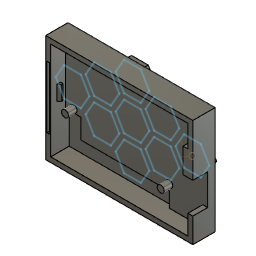
Arduino Pro Holder v8 (Autodesk Fusion 360 design; units mm, degrees)
Autodesk Fusion 360 part; units mm, degrees
sketch "Arduino" plane through (0, 0, 0) normal (0, 0, 1) x (1, 0, 0)
  line L0 (0, 0) -> (54.5, 0)
  line L1 (54.5, 0) -> (54.5, 38.5)
  line L2 (54.5, 38.5) -> (0, 38.5)
  line L3 (0, 38.5) -> (0, 0)
  circle A0 centre (41.5, 8) radius 1.75
  circle A1 centre (2.8, 15) radius 1.75
  line L4 (54.5, 19) -> (48.5, 19)
  line L5 (48.5, 19) -> (48.5, 9)
  line L6 (48.5, 9) -> (54.5, 9)
  line L7 (54.5, 9) -> (54.5, 19)
  dimension "d1" = 54.5
  dimension "d2" = 38.5
  dimension "d3" = 3.5
  dimension "d4" = 3.5
  dimension "d5" = 13
  dimension "d6" = 8
  dimension "d7" = 15
  dimension "d8" = 2.8
  dimension "d9" = 6
  dimension "d10" = 10
  dimension "d11" = 9
  constraint horizontal L0
  constraint vertical L1
  constraint horizontal L2
  constraint vertical L3
  constraint coincident L0.start L3.end
  constraint horizontal L4
  constraint vertical L5
  constraint horizontal L6
  constraint vertical L7
  constraint coincident L1 L4.start
  measures "d1" distance of L0.start L0.end
  measures "d2" distance of L0.start L2.end
  measures "d3" diameter of A0
  measures "d4" diameter of A1
  measures "d5" distance of L1 A0.centre
  measures "d6" distance of L0 A0.centre
  measures "d7" distance of L0 A1.centre
  measures "d8" distance of L3 A1.centre
  measures "d9" distance of L4.start L4.end
  measures "d10" distance of L4.start L6.end
  measures "d11" distance of L0 L6
sketch "Shell Outline" plane through (0, 0, 0) normal (0, 0, 1) x (1, 0, 0)
  circle A0 centre (-0.6853, 15.304) radius 1.4
  circle A1 centre (38.0147, 8.304) radius 1.4
  line L0 (51.5147, 39.304) -> (-3.9853, 39.304)
  line L1 (-3.9853, 39.304) -> (-3.9853, -0.196)
  line L2 (-3.9853, -0.196) -> (51.5147, -0.196)
  line L3 (51.5147, -0.196) -> (51.5147, 39.304)
  line L4 (-5.9853, -2.196) -> (53.5147, -2.196)
  line L5 (53.5147, -2.196) -> (53.5147, 41.304)
  line L6 (53.5147, 41.304) -> (-5.9853, 41.304)
  line L7 (-5.9853, 41.304) -> (-5.9853, -2.196)
  line L8 (51.0147, 20.304) -> (53.5147, 20.304)
  line L9 (53.5147, 20.304) -> (53.5147, 7.804)
  line L10 (53.5147, 7.804) -> (51.0147, 7.804)
  line L11 (51.5147, 39.304) -> (-3.9853, 39.304)
  line L12 (-3.9853, 39.304) -> (-3.9853, 33.304)
  line L13 (-3.9853, 33.304) -> (51.5147, 33.304)
  line L14 (51.5147, 33.304) -> (51.5147, 39.304)
  line L15 (-3.9853, -0.196) -> (38.0147, -0.196)
  line L16 (38.0147, -0.196) -> (38.0147, 5.804)
  line L17 (38.0147, 5.804) -> (-3.9853, 5.804)
  line L18 (-3.9853, 5.804) -> (-3.9853, -0.196)
  line L19 (-3.9853, 5.804) -> (2.259, 5.804)
  line L20 (2.259, 5.804) -> (2.259, 13.804)
  line L21 (2.259, 13.804) -> (-3.9853, 13.804)
  line L22 (-3.9853, 13.804) -> (-3.9853, 5.804)
  point P0 (-3.4853, 0.304)
  dimension "d16" = 2.8
  dimension "d17" = 2.8
  dimension "d33" = 12.5
  dimension "d34" = 8
  dimension "d36" = 2
  dimension "d37" = 6
  dimension "d38" = 42
  dimension "d39" = 6
  dimension "d40" = 8
  constraint horizontal L8
  constraint vertical L9
  constraint coincident L5 L9.end
  constraint horizontal L11
  constraint vertical L12
  constraint horizontal L13
  constraint vertical L14
  constraint horizontal L15
  constraint vertical L16
  constraint horizontal L17
  constraint vertical L18
  constraint horizontal L19
  constraint vertical L20
  constraint horizontal L21
  constraint vertical L22
  measures "d16" diameter of A1
  measures "d17" diameter of A0
  measures "d33" distance of L8 L10
  measures "d34" distance of L2 L10
  measures "d36" distance of L2 L4
  measures "d37" distance of L0.start L13.end
  measures "d38" distance of L1.end L15.end
  measures "d39" distance of L1.end L17.end
  measures "d40" distance of L17.end L21.end
extrude "Extrude1" add sketch "Arduino" along normal blind 6 contours L0 L1 L2 L3 L4 L5 L6 makes body 1
move_body "Move1" bodies 1 to x (1, 0, 0) y (0, 1, 0) z (0, 0, 1) at (-3, 0, 0)
move_body "Move2" bodies 1 to x (1, 0, 0) y (0, 1, 0) z (0, 0, 1) at (-0.4853, 0.304, 0)
extrude "Extrude2" add sketch "Shell Outline" against normal blind 2 separate body contours A0 | A1 | L0 L1 L3 L11 L12 L13 L14 | L0 L1 L2 L3 L4 L5 L6 L7 L8 L10 L11 L12 L14 L15 L18 L22 | L1 L2 L3 L13 L16 L17 L20 L21 | L3 L5 L8 L9 L10 | L1 L17 L19 L20 L21 L22 | L1 L2 L15 L16 L17 L18 L19 makes body 2
extrude "Extrude3" add sketch "Shell Outline" along normal blind 3.5 separate body contours A0 | A1 makes body 3 at (37.9798, 9.7036, 2.3333) makes body 4 at (0.7077, 15.1646, 2.3333)
extrude "Extrude4" add sketch "Shell Outline" along normal blind 6 separate body contours L0 L1 L2 L3 L4 L5 L6 L7 L8 L10 L11 L12 L14 L15 L18 L22 makes body 5
combine "Combine1" operation add target body 2 tool bodies 3 4 5
extrude "Extrude5" cut sketch "Shell Outline" against normal blind 1.5 contours L0 L1 L3 L11 L12 L13 L14 | L1 L17 L19 L20 L21 L22 | L1 L2 L15 L16 L17 L18 L19 bodies 2
extrude "Extrude6" add 1 faces at (33.6814, 26.804, -2) along direction (0, 0, -1) blind 1 on bodies 2 bodies 2
sketch "Sketch3" plane through (51.5147, 0, 0) normal (-1, 0, 0) x (0, 0, 1)
  line L0 (0, 33.304) -> (0, 20.304)
  line L1 (0, 20.304) -> (6, 20.304)
  line L2 (6, 20.304) -> (6, 39.304)
  line L3 (6, 39.304) -> (-1.5, 39.304)
  line L4 (-1.5, 39.304) -> (-1.5, 33.304)
  line L5 (-1.5, 33.304) -> (0, 33.304)
  line L6 (6, 20.304) -> (3, 20.304)
  line L7 (3, 20.304) -> (3, 30.304)
  line L8 (3, 30.304) -> (6, 30.304)
  line L9 (6, 30.304) -> (6, 20.304)
  dimension "d45" = 10
  constraint horizontal L6
  constraint vertical L7
  constraint horizontal L8
  constraint vertical L9
  constraint coincident L1.end L2.start
  measures "d45" distance of L1.end L8.end
extrude "Extrude7" add sketch "Sketch3" along normal blind 2 contours L1 L2 L6 L7 L8 L9 bodies 2
sketch "Sketch4" plane through (-3.9853, 0, 0) normal (1, 0, 0) x (0, 0, -1)
  line L0 (1.5, 39.304) -> (-6, 39.304)
  line L1 (-6, 39.304) -> (-6, -0.196)
  line L2 (-6, -0.196) -> (1.5, -0.196)
  line L3 (1.5, -0.196) -> (1.5, 13.804)
  line L4 (1.5, 13.804) -> (0, 13.804)
  line L5 (0, 13.804) -> (0, 33.304)
  line L6 (0, 33.304) -> (1.5, 33.304)
  line L7 (1.5, 33.304) -> (1.5, 39.304)
  line L8 (-2, 36) -> (-2, 7) construction
  line L9 (-2, 18) -> (-3.5, 18) construction
  line L10 (-3.5, 18) -> (-3.5, 24) construction
  line L11 (-3.5, 24) -> (-2, 24) construction
  line L12 (-2, 24) -> (-2, 18) construction
  line L13 (-3.5, 24) -> (-2, 24)
  line L14 (-2, 24) -> (-2, 18)
  line L15 (-2, 18) -> (-3.5, 18)
  line L16 (-3.5, 18) -> (-3.5, 24)
  dimension "d48" = 2
  dimension "d49" = 1.5
  dimension "d50" = 6
  constraint parallel L5 L8
  constraint horizontal L9
  constraint vertical L10
  constraint horizontal L11
  constraint vertical L12
  constraint coincident L8 L9.start
  constraint horizontal L13
  constraint vertical L14
  constraint horizontal L15
  constraint vertical L16
  measures "d48" distance of L5 L8
  measures "d49" distance of L9.start L9.end
  measures "d50" distance of L9.start L11.end
extrude "Extrude8" add sketch "Sketch4" along normal blind 1 contours L13 L14 L15 L16 bodies 2
chamfer "Chamfer1" distance 1 angle 45 1 edges at (-2.9853, 21, 3.5) on bodies 2
sketch "Sketch5" plane through (0, 0, 6) normal (0, 0, 1) x (1, 0, 0)
  line L0 (49.5147, 20.304) -> (53.5147, 20.304)
  line L1 (53.5147, 20.304) -> (53.5147, 41.304)
  line L2 (53.5147, 41.304) -> (-5.9853, 41.304)
  line L3 (-5.9853, 41.304) -> (-5.9853, -2.196)
  line L4 (-5.9853, -2.196) -> (53.5147, -2.196)
  line L5 (53.5147, -2.196) -> (53.5147, 7.804)
  line L6 (53.5147, 7.804) -> (51.5147, 7.804)
  line L7 (51.5147, 7.804) -> (51.5147, -0.196)
  line L8 (51.5147, -0.196) -> (-3.9853, -0.196)
  line L9 (-3.9853, -0.196) -> (-3.9853, 39.304)
  line L10 (-3.9853, 39.304) -> (51.5147, 39.304)
  line L11 (51.5147, 39.304) -> (51.5147, 30.304)
  line L12 (51.5147, 30.304) -> (49.5147, 30.304)
  line L13 (49.5147, 30.304) -> (49.5147, 20.304)
  line L14 (-5.5, 32.5) -> (-4.5, 32.5)
  line L15 (-4.5, 32.5) -> (-4.5, 7.5)
  line L16 (-4.5, 7.5) -> (-5.5, 7.5)
  line L17 (-5.5, 7.5) -> (-5.5, 32.5)
  dimension "d54" = 1
  dimension "d55" = 25
  constraint horizontal L14
  constraint vertical L15
  constraint horizontal L16
  constraint vertical L17
  measures "d54" distance of L14.start L14.end
  measures "d55" distance of L14.start L16.end
extrude "Extrude9" cut sketch "Sketch5" against normal blind 7 contours L14 L15 L16 L17 bodies 2
sketch "Hex Holder" plane through (0, 0, -3) normal (0, 0, -1) x (-1, 0, 0)
  line L0 (5.9853, 41.304) -> (-53.5147, 41.304)
  line L1 (-53.5147, 41.304) -> (-53.5147, -2.196)
  line L2 (-53.5147, -2.196) -> (5.9853, -2.196)
  line L3 (5.9853, -2.196) -> (5.9853, 41.304)
  line L4 (-37.5724, 19.8127) -> (-40.9643, 25.6877)
  line L5 (-40.9643, 25.6877) -> (-47.7482, 25.6877)
  line L6 (-47.7482, 25.6877) -> (-51.1401, 19.8127)
  line L7 (-51.1401, 19.8127) -> (-47.7482, 13.9377)
  line L8 (-47.7482, 13.9377) -> (-40.9643, 13.9377)
  line L9 (-40.9643, 13.9377) -> (-37.5724, 19.8127)
  line L10 (-44.3563, 19.8127) -> (-39.2684, 16.8752) construction
  line L11 (-44.3563, 19.8127) -> (-39.2684, 22.7502) construction
  line L12 (-39.0158, 12.8127) -> (-35.6238, 6.9377)
  line L13 (-35.6238, 18.6877) -> (-39.0158, 12.8127)
  line L14 (-28.84, 18.6877) -> (-35.6238, 18.6877)
  line L15 (-25.4481, 12.8127) -> (-28.84, 18.6877)
  line L16 (-28.84, 6.9377) -> (-25.4481, 12.8127)
  line L17 (-35.6238, 6.9377) -> (-28.84, 6.9377)
  line L18 (-26.8914, 5.8127) -> (-23.4995, -0.0623)
  line L19 (-23.4995, 11.6877) -> (-26.8914, 5.8127)
  line L20 (-16.7156, 11.6877) -> (-23.4995, 11.6877)
  line L21 (-13.3237, 5.8127) -> (-16.7156, 11.6877)
  line L22 (-16.7156, -0.0623) -> (-13.3237, 5.8127)
  line L23 (-23.4995, -0.0623) -> (-16.7156, -0.0623)
  line L24 (-39.0158, 26.8127) -> (-35.6238, 20.9377)
  line L25 (-35.6238, 32.6877) -> (-39.0158, 26.8127)
  line L26 (-28.84, 32.6877) -> (-35.6238, 32.6877)
  line L27 (-25.4481, 26.8127) -> (-28.84, 32.6877)
  line L28 (-28.84, 20.9377) -> (-25.4481, 26.8127)
  line L29 (-35.6238, 20.9377) -> (-28.84, 20.9377)
  line L30 (-26.8914, 19.8127) -> (-23.4995, 13.9377)
  line L31 (-23.4995, 25.6877) -> (-26.8914, 19.8127)
  line L32 (-16.7156, 25.6877) -> (-23.4995, 25.6877)
  line L33 (-13.3237, 19.8127) -> (-16.7156, 25.6877)
  line L34 (-16.7156, 13.9377) -> (-13.3237, 19.8127)
  line L35 (-23.4995, 13.9377) -> (-16.7156, 13.9377)
  line L36 (-14.7671, 12.8127) -> (-11.3751, 6.9377)
  line L37 (-11.3751, 18.6877) -> (-14.7671, 12.8127)
  line L38 (-4.5913, 18.6877) -> (-11.3751, 18.6877)
  line L39 (-1.1993, 12.8127) -> (-4.5913, 18.6877)
  line L40 (-4.5913, 6.9377) -> (-1.1993, 12.8127)
  line L41 (-11.3751, 6.9377) -> (-4.5913, 6.9377)
  line L42 (-26.8914, 33.8127) -> (-23.4995, 27.9377)
  line L43 (-23.4995, 39.6877) -> (-26.8914, 33.8127)
  line L44 (-16.7156, 39.6877) -> (-23.4995, 39.6877)
  line L45 (-13.3237, 33.8127) -> (-16.7156, 39.6877)
  line L46 (-16.7156, 27.9377) -> (-13.3237, 33.8127)
  line L47 (-23.4995, 27.9377) -> (-16.7156, 27.9377)
  line L48 (-14.7671, 26.8127) -> (-11.3751, 20.9377)
  line L49 (-11.3751, 32.6877) -> (-14.7671, 26.8127)
  line L50 (-4.5913, 32.6877) -> (-11.3751, 32.6877)
  line L51 (-1.1993, 26.8127) -> (-4.5913, 32.6877)
  line L52 (-4.5913, 20.9377) -> (-1.1993, 26.8127)
  line L53 (-11.3751, 20.9377) -> (-4.5913, 20.9377)
  line L54 (-2.6427, 19.8127) -> (0.7492, 13.9377)
  line L55 (0.7492, 25.6877) -> (-2.6427, 19.8127)
  line L56 (7.5331, 25.6877) -> (0.7492, 25.6877)
  line L57 (10.925, 19.8127) -> (7.5331, 25.6877)
  line L58 (7.5331, 13.9377) -> (10.925, 19.8127)
  line L59 (0.7492, 13.9377) -> (7.5331, 13.9377)
  point P0 (-44.3563, 19.8127)
  dimension "d64" = 11.75
  dimension "d67" = 14
  dimension "d68" = 14
  constraint coincident P0 L10.start
  constraint midpoint L9 L10.end
  constraint midpoint L4 L11.end
  measures "d64" distance of L4 L7
extrude "Extrude10" add sketch "Hex Holder" along normal blind 3 contours L4 L5 L6 L7 L8 L9 | L36 L37 L38 L39 L40 L41 | L42 L43 L44 L45 L46 L47 bodies 2
hidden bodies 1
named bodies: "Arduino"
